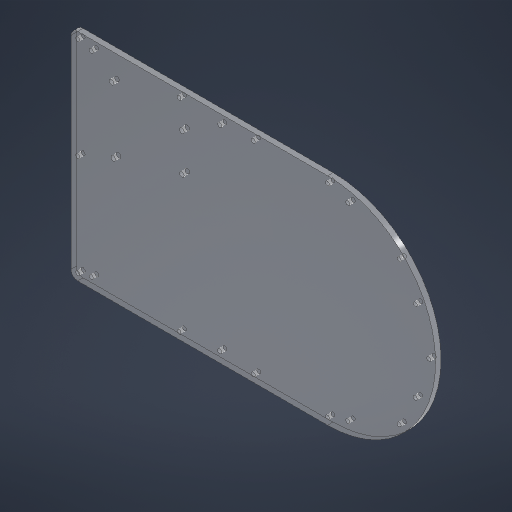
# Autodesk Inventor part: testbasedown
Saved by Autodesk Inventor 2025.2 (Build 292293000, 293)
## iProperties
Created: 2025-04-27
Part Number: testbasedown
Material: Generic
Document SubType Name: Modeling
Designer: Tiago
Density: 1 g/cm^3
Appearance: Polycarbonate - Clear
Mass: 159.889 g
Surface Area: 836.081 cm^2
Volume: 159.889 cm^3
Author: Tiago
Autodesk Inventor part; units mm, degrees
ref_plane "YZ Plane" through (0, 0, 0) normal (1, 0, 0) x (0, 1, 0)
ref_plane "XZ Plane" through (0, 0, 0) normal (0, 1, 0) x (-1, 0, 0)
ref_plane "XY Plane" through (0, 0, 0) normal (0, 0, 1) x (1, 0, 0)
sketch "Sketch1" plane through (0, 0, 0) normal (0, 0, 1) x (1, 0, 0)
  line L0 (-185, -80) -> (0, -80)
  line L1 (0, 80) -> (-185, 80)
  line L2 (-190, 75) -> (-190, -75)
  line L3 (80, 0) -> (80, 0)
  arc A0 (0, -80) -> (80, 0) centre (0, 0) ccw
  arc A1 (80, 0) -> (0, 80) centre (0, 0) ccw
  circle A2 centre (75, 0) radius 1.5
  circle A3 centre (53.033, -53.033) radius 1.5
  circle A4 centre (0, -75) radius 1.5
  circle A5 centre (-55, -75) radius 1.5
  circle A6 centre (-110, -75) radius 1.5
  circle A7 centre (-185, -75) radius 1.5
  circle A8 centre (-185, 0) radius 1.5
  circle A9 centre (53.033, 53.033) radius 1.5
  circle A10 centre (0, 75) radius 1.5
  circle A11 centre (-55, 75) radius 1.5
  circle A12 centre (-110, 75) radius 1.5
  circle A13 centre (-185, 75) radius 1.5
  circle A14 centre (65, -30) radius 1.5
  circle A15 centre (65, 30) radius 1.5
  circle A16 centre (15, -70) radius 1.5
  circle A17 centre (-175, -72.5) radius 1.5
  circle A18 centre (-80, -72.5) radius 1.5
  circle A19 centre (15, 70) radius 1.5
  circle A20 centre (-175, 72.5) radius 1.5
  circle A21 centre (-80, 72.5) radius 1.5
  circle A22 centre (-160, 60) radius 1.75
  circle A23 centre (-158.73, 11.74) radius 1.75
  circle A24 centre (-107.93, 54.92) radius 1.75
  circle A25 centre (-107.93, 26.98) radius 1.75
  arc A26 (-185, 80) -> (-190, 75) centre (-185, 75) ccw
  arc A27 (-190, -75) -> (-185, -80) centre (-185, -75) ccw
  point P0 (120, -80)
  point P1 (80, 0)
  point P2 (-190, 0)
  point P3 (-92.5, -80)
  dimension "d49" = 80
  dimension "Furos" = 3
  dimension "d55" = 3
  dimension "d57" = 3
  dimension "d61" = 3
  dimension "d62" = 3
  dimension "d63" = 3
  dimension "d64" = 3
  dimension "d71" = 3
  dimension "d75" = 3
  dimension "d79" = 3
  dimension "d84" = 3
  dimension "d87" = 3.5
  dimension "d89" = 3.5
  dimension "d97" = 3.5
  dimension "d99" = 3.5
  dimension "d107" = 80
  dimension "d108" = 80
  dimension "d109" = 160
  dimension "d110" = 190
  dimension "d111" = 80
  dimension "d112" = 80
  dimension "d113" = 75
  dimension "d114" = 5
  dimension "d115" = 30
  dimension "d116" = 65
  dimension "d117" = 53.033
  dimension "d118" = 53.033
  dimension "d119" = 70
  dimension "d120" = 15
  dimension "d121" = 75
  dimension "d122" = 31.27
  dimension "d123" = 30
  dimension "d124" = 20
  dimension "d125" = 68.26
  dimension "d126" = 25.08
  dimension "d128" = 82.07
  dimension "d129" = 82.07
  dimension "d130" = 5
  dimension "d131" = 75
  dimension "d132" = 75
  dimension "d133" = 3
  dimension "d134" = 3
  dimension "d135" = 3
  dimension "d136" = 30
  dimension "d137" = 53.033
  dimension "d138" = 70
  dimension "d139" = 72.5
  dimension "d141" = 55
  dimension "d142" = 110
  dimension "d143" = 75
  dimension "d145" = 3
  dimension "d146" = 3
  dimension "d147" = 107.93
  dimension "d148" = 3
  dimension "d149" = 5
  dimension "d150" = 7.5
  dimension "d151" = 3
  dimension "d152" = 3
  dimension "d153" = 7.5
  dimension "d154" = 15
  dimension "d155" = 95
  dimension "d156" = 5
  dimension "d157" = 5
  constraints: 28 centre point, 12 vertical alignment, 8 coincident, 8 end point, 8 horizontal alignment, 8 point on circle, 4 tangent, 2 midpoint, 1 concentric, 1 horizontal, 1 parallel, 1 perpendicular
  measures "d49" radius of A0
  measures "Furos" diameter of A2
  measures "d55" diameter of A3
  measures "d57" diameter of A4
  measures "d61" diameter of A5
  measures "d62" diameter of A6
  measures "d63" diameter of A7
  measures "d64" diameter of A8
  measures "d71" diameter of A14
  measures "d75" diameter of A16
  measures "d79" diameter of A17
  measures "d84" diameter of A18
  measures "d87" diameter of A22
  measures "d89" diameter of A23
  measures "d97" diameter of A24
  measures "d99" diameter of A25
  measures "d107" distance from line of L0 A0.centre
  measures "d108" distance from line of L1 A0.centre
  measures "d109" distance between parallel lines of L0 L1
  measures "d110" distance from line of A0.centre L2
  measures "d111" distance of L3.start A0.centre
  measures "d112" radius of A1
  measures "d113" distance of A0.centre A2.centre
  measures "d114" distance of L3.end A2.centre
  measures "d115" vertical distance of A0.centre A15.centre
  measures "d116" horizontal distance of A0.centre A15.centre
  measures "d117" horizontal distance of A1.centre A9.centre
  measures "d118" horizontal distance of A9.centre A0.centre
  measures "d119" vertical distance of A0.centre A19.centre
  measures "d120" horizontal distance of A19.centre A0.centre
  measures "d121" distance of A1.centre A10.centre
  measures "d122" distance from line of L2 A23.centre
  measures "d123" distance from line of L2 A22.centre
  measures "d124" distance from line of L1 A22.centre
  measures "d125" distance from line of L1 A23.centre
  measures "d126" distance from line of L1 A24.centre
  measures "d128" distance from line of L2 A25.centre
  measures "d129" distance from line of L2 A24.centre
  measures "d130" distance of point (-190, 0) A8.centre
  measures "d131" distance of point (0, 0) A4.centre
  measures "d132" distance of A0.centre A10.centre
  measures "d133" diameter of A10
  measures "d134" diameter of A19
  measures "d135" diameter of A9
  measures "d136" vertical distance of point (0, 0) A14.centre
  measures "d137" horizontal distance of point (0, 0) A3.centre
  measures "d138" vertical distance of point (0, 0) A16.centre
  measures "d139" vertical distance of point (0, 0) A18.centre
  measures "d141" horizontal distance of point (0, 0) A5.centre
  measures "d142" horizontal distance of A0.centre A6.centre
  measures "d143" vertical distance of point (0, 0) A6.centre
  measures "d145" diameter of A20
  measures "d146" diameter of A12
  measures "d147" horizontal distance of point (0, 0) A24.centre
  measures "d148" diameter of A13
  measures "d149" distance from line of L2 A13.centre
  measures "d150" distance from line of L1 A20.centre
  measures "d151" diameter of A11
  measures "d152" diameter of A21
  measures "d153" distance from line of L1 A21.centre
  measures "d154" distance from line of L2 A17.centre
  measures "d155" distance of A17.centre A18.centre
  measures "d156" radius of A26
  measures "d157" distance from line of L2 L1.end
extrude "Extrusion1" add sketch "Sketch1" along normal blind 4
equation "\"d55\" = Furos"
equation "\"d57\" = Furos"
equation "\"d61\" = Furos"
equation "\"d62\" = Furos"
equation "\"d63\" = Furos"
equation "\"d64\" = Furos"
equation "\"d71\" = FA"
equation "\"d75\" = FA"
equation "\"d79\" = FA"
equation "\"d84\" = FA"
equation "\"FA\" = 3"
body "Solid1"
